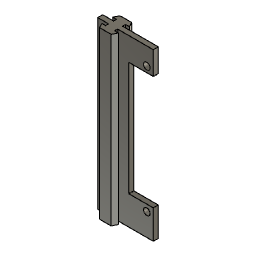
PCB mount v5 (Autodesk Fusion 360 design; units mm, degrees)
Autodesk Fusion 360 part; units mm, degrees
sketch "Sketch1" plane through (0, 0, 0) normal (0, 0, 1) x (1, 0, 0)
  line L0 (-1.4695, 2.841) -> (8.5305, 2.841)
  line L1 (8.5305, 2.841) -> (7.0305, -0.059)
  line L2 (0.7805, 2.841) -> (6.25, 2.841)
  line L3 (6.25, 2.841) -> (6.25, 4.641)
  line L4 (0.7805, 4.641) -> (0.7805, 2.841)
  line L5 (0.7805, 4.641) -> (-5.75, 4.641)
  line L6 (-5.75, 4.641) -> (-5.75, 6.141)
  line L7 (0.7805, 6.141) -> (0.7805, 4.641)
  line L8 (6.25, 4.641) -> (12.75, 4.641)
  line L9 (12.75, 4.641) -> (12.75, 6.141)
  line L10 (6.25, 6.141) -> (6.25, 4.641)
  line L11 (6.25, 6.141) -> (6.25, 4.641)
  line L12 (6.25, 4.641) -> (0.7805, 4.641)
  line L13 (0.7805, 4.641) -> (0.7805, 6.141)
  line L14 (-8.5568, 6.141) -> (16.5, 6.141)
  line L15 (8.5305, 9.441) -> (7.0305, 12.341)
  line L16 (6.25, 9.441) -> (6.25, 7.641)
  line L17 (6.25, 6.141) -> (6.25, 7.641)
  line L18 (-1.4695, 9.441) -> (8.5305, 9.441)
  line L19 (0.7805, 7.641) -> (-5.75, 7.641)
  line L20 (6.25, 6.141) -> (6.25, 7.641)
  line L21 (12.75, 7.641) -> (12.75, 6.141)
  line L22 (6.25, 7.641) -> (12.75, 7.641)
  line L23 (0.0305, 12.341) -> (7.0305, 12.341)
  line L24 (0.7805, 6.141) -> (0.7805, 7.641)
  line L25 (0.7805, 9.441) -> (6.25, 9.441)
  line L26 (6.25, 7.641) -> (0.7805, 7.641)
  line L27 (0.7805, 7.641) -> (0.7805, 9.441)
  line L28 (-5.75, 7.641) -> (-5.75, 6.141)
  line L29 (0.7805, 7.641) -> (0.7805, 6.141)
  line L30 (-1.4695, 2.841) -> (0.0305, -0.059)
  line L31 (0.0305, -0.059) -> (7.0305, -0.059)
  line L32 (0.0305, 12.341) -> (-1.4695, 9.441)
  point P0 (0.0305, -0.059)
  point P1 (7.0305, -0.059)
  point P2 (8.5305, 2.841)
  point P3 (-1.4695, 2.841)
  point P4 (6.2805, 2.841)
  point P5 (0.7805, 2.841)
  point P6 (0.0305, 12.341)
  point P7 (-1.4695, 9.441)
  point P8 (6.2805, 9.441)
  point P9 (0.7805, 9.441)
  point P10 (0, 12.282)
  point P11 (0, 12.282)
  point P12 (7.0305, 12.341)
  point P13 (8.5305, 9.441)
  dimension "d1" = 7
  dimension "d2" = 10
  dimension "d4" = 5.5
  dimension "d5" = 2.25
  dimension "d6" = 1.8
  dimension "d7" = 6.5
  dimension "d8" = 1.5
  dimension "d12" = 1.8
  constraint horizontal P0 L1.end
  constraint horizontal P2 L0.start
  constraint coincident P3 L0.start
  constraint coincident P2 L0.end
  constraint coincident P1 L1.end
  constraint coincident L0 P4
  constraint coincident L0 P5
  constraint horizontal L2
  constraint vertical L3
  constraint vertical L4
  constraint coincident P5 L2.start
  constraint horizontal L5
  constraint vertical L6
  constraint vertical L7
  constraint horizontal L8
  constraint vertical L9
  constraint vertical L10
  constraint vertical L11
  constraint horizontal L12
  constraint vertical L13
  constraint perpendicular L6 L14
  constraint symmetric origin L14 P11
  constraint symmetric P0 L14 P6
  constraint symmetric P1 L14 P12
  constraint symmetric P2 L14 P13
  constraint symmetric P3 L14 P7
  constraint symmetric P4 L14 P8
  constraint symmetric P5 L14 P9
  constraint symmetric L2.end L14 L16.start
  constraint symmetric L3.end L14 L16.end
  constraint symmetric L4.start L14 L19.start
  constraint symmetric L5.end L14 L19.end
  constraint symmetric L6.end L14 L28.end
  constraint symmetric L7.start L14 L13.end
  constraint symmetric L8.end L14 L21.start
  constraint symmetric L9.end L14 L21.end
  constraint symmetric L10.start L14 L11.start
  constraint coincident P0 L30.end
  measures "d1" distance of P0 L1.end
  measures "d2" distance of P2 L0.start
  measures "d4" distance of P4 P5
  measures "d5" distance of P3 P5
  measures "d6" distance of P5 L4.start
  measures "d7" distance of L3.end L8.end
  measures "d8" distance of L3.end L10.start
  measures "d12" distance of L0 L8
extrude "Extrude2" add sketch "Sketch1" along normal blind 10
extrude "Extrude3" add 1 faces at (4.437, 0.9077, 10) along direction (0, 0, 1) blind 15
extrude "Extrude4" add 1 faces at (12.75, 5.641, 8.3333) along direction (1, 0, 0) blind 15
sketch "Sketch2" plane through (0, 7.641, 0) normal (0, 1, 0) x (-1, 0, 0)
  line L0 (-27.75, 0) -> (-6.25, 0)
  line L1 (-6.25, 0) -> (-6.25, 25)
  line L2 (-6.25, 25) -> (-27.75, 25)
  line L3 (-27.75, 25) -> (-27.75, 0)
  line L4 (-8.5305, 0, 1.8) -> (-8.5305, 25, 1.8)
  point P0 (-23.8463, 13.4874)
  dimension "d19" = 13.5
  dimension "d20" = 15.5
  measures "d19" distance of L0 P0
extrude "Extrude5" cut 1 faces at (13.4167, 5.641, 25) along direction (0, 0, -1) blind 7
extrude "Extrude6" cut 1 faces at (27.75, 5.641, 6) along direction (-1, 0, 0) blind 4
extrude "Extrude7" add 1 faces at (23.75, 5.641, 6) along direction (1, 0, 0) blind 8
hole "Hole2" at (23.8463, 7.0585, 13.4874) direction (0, -1, 0) diameter 4 depth 8 tip angle 180
extrude "Extrude8" cut 1 faces at (23.1941, 7.0585, 12.9987) along direction (0, 1, 0) blind 2
extrude "Extrude9" cut 1 faces at (31.75, 5.641, 6) along direction (-1, 0, 0) blind 2
extrude "Extrude10" add 1 faces at (14.0833, 5.641, 18) along direction (0, 0, 1) blind 80
extrude "Extrude11" add 1 faces at (14.0833, 5.641, 98) along direction (0, 0, 1) blind 1
sketch "Sketch3" plane through (0, 7.641, 0) normal (0, 1, 0) x (-1, 0, 0)
  line L0 (-29.75, 99) -> (-29.75, 0)
  line L1 (-29.75, 0) -> (-6.25, 0)
  line L2 (-6.25, 0) -> (-6.25, 99)
  line L3 (-6.25, 99) -> (-29.75, 99)
  circle A0 centre (-23.8463, 13.4874) radius 2
  point P0 (-23.8296, 89.4874)
  dimension "d41" = 76
  measures "d41" distance of A0.centre P0
hole "Hole3" at (23.8296, 7.641, 89.4874) direction (0, -1, 0) diameter 4 depth 6 tip angle 180
extrude "Extrude12" add 1 faces at (14.0833, 5.641, 99) along direction (0, 0, 1) blind 1
extrude "Extrude13" cut 1 faces at (29.75, 6.641, 33.3333) along direction (-1, 0, 0) blind 2
sketch "Sketch4" plane through (0, 7.641, 0) normal (0, 1, 0) x (-1, 0, 0)
  line L0 (-28, 86) -> (-13, 86)
  line L1 (-13, 86) -> (-13, 17.4372)
  line L2 (-13, 17.4372) -> (-28, 17.4372)
  line L3 (-28, 17.4372) -> (-28, 86)
  constraint horizontal L0
  constraint vertical L1
  constraint horizontal L2
  constraint vertical L3
extrude "Extrude14" cut sketch "Sketch4" against normal blind 3
